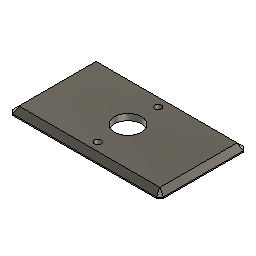
COMPACT_ROBOT_G2 v1 (Autodesk Fusion 360 design; units mm, degrees)
Autodesk Fusion 360 part; units mm, degrees
sketch "Esboço1" plane through (0, 0, 0) normal (0, 0, 1) x (1, 0, 0)
  line L0 (91, 75) -> (134, 75)
  line L1 (135, 74.006) -> (135, 50)
  line L2 (134.006, 49) -> (91, 49)
  line L3 (90, 49.994) -> (90, 74.006)
  line L4 (134, 75) -> (135, 74.006)
  line L5 (134, 75) -> (134, 49) construction
  line L6 (135, 74.006) -> (90, 74.006) construction
  line L7 (135, 50) -> (90, 50) construction
  line L8 (91, 49) -> (91, 75) construction
  line L9 (135, 50) -> (134.006, 49)
  line L10 (91, 49) -> (90, 49.994)
  line L11 (91, 75) -> (90, 74.006)
  circle A0 centre (112.503, 62) radius 4
  line L12 (90, 62) -> (135, 62.003) construction
  circle A1 centre (112.503, 71) radius 1
  circle A2 centre (112.5042, 53.003) radius 1
  point P0 (90, 75)
  point P1 (135, 75)
  point P2 (135, 49)
  point P3 (90, 49)
  dimension "d20" = 26
  dimension "d21" = 45
  dimension "d22" = 1
  dimension "d24" = 1.41
  dimension "d25" = 1
  dimension "d28" = 1.41
  dimension "d29" = 1
  dimension "d31" = 1.41
  dimension "d32" = 1
  dimension "d34" = 1.41
  dimension "d35" = 8
  dimension "d36" = 2
  dimension "d37" = 9
  constraint horizontal L0
  constraint vertical L1
  constraint horizontal L2
  constraint vertical L3
  constraint coincident P1 L0
  constraint coincident P1 L1
  constraint coincident L2 L5.end
  constraint coincident L3 L6.end
  constraint coincident L1 L7.start
  constraint coincident L3 L7.end
  constraint perpendicular L3 L7
  constraint coincident L2 L8.start
  constraint coincident L0 L8.end
  constraint perpendicular L0 L8
  constraint coincident P2 L1
  constraint coincident P2 L2
  constraint coincident P3 L2
  constraint coincident P3 L3
  constraint coincident P0 L0
  constraint coincident P0 L3
  constraint midpoint L3 L12.start
  constraint midpoint L1 L12.end
  constraint symmetric L12 A1 A2
  measures "d20" distance of P0 P3
  measures "d21" distance of P2 P3
  measures "d22" distance of P1 L0.end
  measures "d24" distance of L0.end L1.start
  measures "d25" distance of P2 L1.end
  measures "d28" distance of L1.end L2.start
  measures "d29" distance of P3 L2.end
  measures "d31" distance of L2.end L3.start
  measures "d32" distance of P0 L0.start
  measures "d34" distance of L0.start L3.end
  measures "d35" diameter of A0
  measures "d36" diameter of A1
  measures "d37" distance of A0.centre A1.centre
extrude "Extrusão2" add sketch "Esboço1" along normal blind 1.85
chamfer "Chanfro2" distance 1.5 angle 45 8 edges at (112.503, 49, 1.85) (90.5, 49.497, 1.85) (134.503, 49.5, 1.85) (135, 62.003, 1.85) (134.5, 74.503, 1.85) (112.5, 75, 1.85) (90.5, 74.503, 1.85) (90, 62, 1.85)
